feet v1 (Autodesk Fusion 360 design; units mm, degrees)
Autodesk Fusion 360 part; units mm, degrees
note: some values were not read from the file. Set by a fixed rule: which sketch regions a step uses.
sketch "Sketch1" plane through (0, 0, 0) normal (0, 0, 1) x (1, 0, 0)
  line L0 (160, -67.5) -> (-160, -67.5)
  line L1 (-160, -67.5) -> (-160, 67.5)
  line L2 (-160, 67.5) -> (160, 67.5)
  line L3 (160, 67.5) -> (160, -67.5)
  line L4 (160, -67.5) -> (-160, 67.5) construction
  line L5 (-160, -67.5) -> (160, 67.5) construction
  line L6 (-160, 67.5) -> (-125, 67.5)
  line L7 (-125, 67.5) -> (-125, 42.5)
  line L8 (-125, 42.5) -> (-160, 42.5)
  line L9 (-160, 42.5) -> (-160, 67.5)
  line L10 (125, 42.5) -> (160, 42.5)
  line L11 (160, 42.5) -> (160, 67.5)
  line L12 (160, 67.5) -> (125, 67.5)
  line L13 (125, 67.5) -> (125, 42.5)
  dimension "d1" = 320
  dimension "d2" = 135
  dimension "d3" = 35
  dimension "d4" = 35
  dimension "d5" = 25
  dimension "d6" = 25
  constraint horizontal L0
  constraint perpendicular L0 L1
  constraint parallel L0 L2
  constraint parallel L1 L3
  constraint coincident L4 origin
  constraint coincident L5 origin
  constraint horizontal L6
  constraint vertical L7
  constraint horizontal L8
  constraint vertical L9
  constraint horizontal L10
  constraint vertical L11
  constraint horizontal L12
  constraint vertical L13
  measures "d1" distance of L1.end L2.end
  measures "d2" distance of L0.end L1.end
  measures "d3" distance of L7.end L8.end
  measures "d4" distance of L10.start L10.end
  measures "d5" distance of L10.start L12.end
  measures "d6" distance of L6.end L7.end
extrude "Extrude1" add sketch "Sketch1" along normal blind 20
sketch "Sketch2" plane through (0, 0, 20) normal (0, 0, 1) x (1, 0, 0)
  line L0 (160, -67.5) -> (160, 67.5)
  line L1 (160, 67.5) -> (-160, 67.5)
  line L2 (-160, 67.5) -> (-160, -67.5)
  line L3 (-160, -67.5) -> (160, -67.5)
  line L4 (-125, 35.633) -> (125, 35.633)
  dimension "d9" = 250
  dimension "d11" = 103.133
  measures "d9" distance of L4.start L4.end
  measures "d11" distance of L3 L4
hole "Hole1" at (-125, 35.633, 20) at (125, 35.633, 20) direction (0, 0, -1) diameter 30 depth 50 tip angle 118
sketch "Sketch3" plane through (0, 0, 20) normal (0, 0, 1) x (1, 0, 0)
  circle A0 centre (-125, 35.633) radius 15
  circle A1 centre (125, 35.633) radius 15
  line L0 (160, -67.5) -> (160, 67.5)
  line L1 (160, 67.5) -> (-160, 67.5)
  line L2 (-160, 67.5) -> (-160, -67.5)
  line L3 (-160, -67.5) -> (160, -67.5)
  line L4 (-125, 35.633) -> (-160, 35.633)
  line L5 (125, 35.633) -> (126.752, 35.633)
  line L6 (126.752, 35.633) -> (160, 35.633)
  line L7 (125, 35.633) -> (90, 35.633)
  line L8 (-125, 35.633) -> (-90, 35.633)
  line L9 (-90, 35.633) -> (-90, -19.367)
  line L10 (90, 35.633) -> (90, -19.367)
  line L11 (-90, -19.367) -> (90, -19.367)
  line L12 (-125, 35.633) -> (-125, 67.5)
  line L13 (125, 35.633) -> (125, 67.5)
  arc A2 (-90, 35.633) -> (-160, 35.633) centre (-125, 32.346) ccw
  arc A3 (160, 35.633) -> (90, 35.633) centre (125, 32.346) ccw
  dimension "d15" = 55
  dimension "d16" = 70
  dimension "d17" = 55
  constraint coincident A0.centre L4.start
  constraint coincident L2 L4.end
  constraint perpendicular L2 L4
  constraint coincident A1.centre L5.start
  constraint parallel L4 L5
  constraint coincident L0 L6.end
  constraint perpendicular L0 L6
  constraint perpendicular L0 L7
  constraint parallel L4 L8
  constraint perpendicular L4 L9
  constraint perpendicular L7 L10
  constraint coincident L1 L12.end
  constraint perpendicular L1 L12
  constraint coincident L1 L13.end
  constraint perpendicular L1 L13
  constraint coincident L12.end A2
  constraint coincident L13.end A3
  constraint tangent L1 A3
  measures "d15" distance of L8.end L9.end
  measures "d16" distance of L2 L9
  measures "d17" distance of L7.end L10.end
extrude "Extrude2" cut sketch "Sketch3" against normal blind 20 contours L1 L9 L10 L11 A2 A3 | L1 L2 A2 | L0 L1 A3
sketch "Sketch4" plane through (0, -19.367, 0) normal (0, 1, 0) x (-1, 0, 0)
  line L0 (90, 20) -> (-90, 20)
  line L1 (-90, 20) -> (-90, 0)
  line L2 (-90, 0) -> (90, 0)
  line L3 (90, 0) -> (90, 20)
  line L4 (90, 10) -> (65, 10)
  line L5 (-90, 10) -> (-65, 10)
  line L6 (0, 10) -> (-25, 10)
  dimension "d20" = 25
  dimension "d21" = 25
  dimension "d22" = 10
  dimension "d23" = 10
  dimension "d24" = 25
  dimension "d25" = 10
  constraint midpoint L3 L4.start
  constraint perpendicular L3 L4
  constraint horizontal L5
  constraint parallel L2 L6
  measures "d20" distance of L6.start L6.end
  measures "d21" distance of L5.start L5.end
  measures "d22" distance of L0 L5
  measures "d23" distance of L2 L6
  measures "d24" distance of L4.start L4.end
  measures "d25" distance of L2 L4
hole "Hole2" at (-65, -19.367, 10) at (0, -19.367, 10) at (65, -19.367, 10) direction (0, -1, 0) diameter 8.5 end through all
fillet "Fillet1" radius 16 2 edges at (-90, -19.367, 10) (90, -19.367, 10)
chamfer "Chamfer1" distance 2 angle 45 18 edges at (-125, 67.5, 20) (-90, 16.133, 20) (90, 16.133, 20) (85.3137, -14.6807, 20) (0, -19.367, 20) (-85.3137, -14.6807, 20) (125, 67.5, 20) (160, -15.9335, 20) (-160, -15.9335, 20) (160, -15.9335, 0) (125, 67.5, 0) (90, 16.133, 0) (-90, 16.133, 0) (-85.3137, -14.6807, 0) (0, -19.367, 0) (85.3137, -14.6807, 0) (-125, 67.5, 0) (-160, -15.9335, 0)
equation "d2 = 160 mm - 25 mm"
equation "d9 = 320 mm - 35 mm - 35 mm"
equation "d11 = 88.133 mm + 15 mm"
